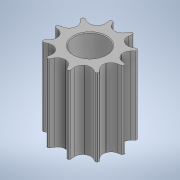
# Autodesk Inventor part: Pulley HTD 3M 10T
Saved by Autodesk Inventor 2022.2 (Build 262287030, 287C)
## iProperties
Created: 2019-06-06
Part Number: Pulley HTD 3M 10T
Material: Generic
Description: STEP AP214
Document SubType Name: Modeling
Designer: Jochen
Density: 1 g/cm^3
Appearance: Default(2)
Sending System: PARTsolutions
Title: C:/Users/StangenbergN/Desktop/Steps Zahnriemenräder/K166_HTD-Zahnwellen/17091100.stp
Revision Number: NONE
Autodesk Inventor part; units mm, degrees
ref_plane "YZ Plane" through (0, 0, 0) normal (1, 0, 0) x (0, 1, 0)
ref_plane "XZ Plane" through (0, 0, 0) normal (0, 1, 0) x (-1, 0, 0)
ref_plane "XY Plane" through (0, 0, 0) normal (0, 0, 1) x (1, 0, 0)
sketch "Sketch3" plane through (0, 0, 0) normal (0, 1, 0) x (-1, 0, 0)
  line L0 (0.8939, 3.7122) -> (1.1141, 4.1058)
  arc A0 (1.3267, 4.19) -> (1.1141, 4.1058) centre (1.272, 4.0174) ccw
  arc A1 (1.3895, 4.1696) -> (1.3267, 4.19) centre (0, 0) ccw
  arc A2 (1.512, 3.9765) -> (1.3895, 4.1696) centre (1.3323, 3.9979) ccw
  line L1 (1.512, 3.9765) -> (1.4588, 3.5286)
  arc A3 (1.4588, 3.5286) -> (1.8604, 2.6099) centre (2.4429, 3.4117) ccw
  line L2 (1.8604, 2.6099) -> (1.9073, 2.5759)
  arc A4 (1.9073, 2.5759) -> (2.9051, 2.4778) centre (2.4898, 3.3776) ccw
  line L3 (2.9051, 2.4778) -> (3.3146, 2.6668)
  arc A5 (3.5361, 2.61) -> (3.3146, 2.6668) centre (3.3905, 2.5025) ccw
  arc A6 (3.5749, 2.5565) -> (3.5361, 2.61) centre (0, 0) ccw
  arc A7 (3.5606, 2.3283) -> (3.5749, 2.5565) centre (3.4277, 2.4512) ccw
  line L4 (3.5606, 2.3283) -> (3.2543, 1.9972)
  arc A8 (3.2543, 1.9972) -> (3.0392, 1.018) centre (3.9817, 1.3242) ccw
  line L5 (3.0392, 1.018) -> (3.0571, 0.9628)
  arc A9 (3.0571, 0.9628) -> (3.8067, 0.297) centre (3.9996, 1.2691) ccw
  line L6 (3.8067, 0.297) -> (4.2491, 0.2092)
  arc A10 (4.3949, 0.033) -> (4.2491, 0.2092) centre (4.2139, 0.0317) ccw
  arc A11 (4.3949, -0.033) -> (4.3949, 0.033) centre (0, 0) ccw
  arc A12 (4.2491, -0.2092) -> (4.3949, -0.033) centre (4.2139, -0.0317) ccw
  line L7 (4.2491, -0.2092) -> (3.8067, -0.297)
  arc A13 (3.8067, -0.297) -> (3.0571, -0.9628) centre (3.9996, -1.2691) ccw
  line L8 (3.0571, -0.9628) -> (3.0392, -1.018)
  arc A14 (3.0392, -1.018) -> (3.2543, -1.9972) centre (3.9817, -1.3242) ccw
  line L9 (3.2543, -1.9972) -> (3.5606, -2.3283)
  arc A15 (3.5749, -2.5565) -> (3.5606, -2.3283) centre (3.4277, -2.4512) ccw
  arc A16 (3.5361, -2.61) -> (3.5749, -2.5565) centre (0, 0) ccw
  arc A17 (3.3146, -2.6668) -> (3.5361, -2.61) centre (3.3905, -2.5025) ccw
  line L10 (3.3146, -2.6668) -> (2.9051, -2.4778)
  arc A18 (2.9051, -2.4778) -> (1.9073, -2.5759) centre (2.4898, -3.3776) ccw
  line L11 (1.9073, -2.5759) -> (1.8604, -2.6099)
  arc A19 (1.8604, -2.6099) -> (1.4588, -3.5286) centre (2.4429, -3.4117) ccw
  line L12 (1.4588, -3.5286) -> (1.512, -3.9765)
  arc A20 (1.3895, -4.1696) -> (1.512, -3.9765) centre (1.3323, -3.9979) ccw
  arc A21 (1.3267, -4.19) -> (1.3895, -4.1696) centre (0, 0) ccw
  arc A22 (1.1141, -4.1058) -> (1.3267, -4.19) centre (1.272, -4.0174) ccw
  line L13 (1.1141, -4.1058) -> (0.8939, -3.7122)
  arc A23 (0.8939, -3.7122) -> (0.029, -3.205) centre (0.029, -4.196) ccw
  line L14 (0.029, -3.205) -> (-0.029, -3.205)
  arc A24 (-0.029, -3.205) -> (-0.8939, -3.7122) centre (-0.029, -4.196) ccw
  line L15 (-0.8939, -3.7122) -> (-1.1141, -4.1058)
  arc A25 (-1.3267, -4.19) -> (-1.1141, -4.1058) centre (-1.272, -4.0174) ccw
  arc A26 (-1.3895, -4.1696) -> (-1.3267, -4.19) centre (0, 0) ccw
  arc A27 (-1.512, -3.9765) -> (-1.3895, -4.1696) centre (-1.3323, -3.9979) ccw
  line L16 (-1.512, -3.9765) -> (-1.4588, -3.5286)
  arc A28 (-1.4588, -3.5286) -> (-1.8604, -2.6099) centre (-2.4429, -3.4117) ccw
  line L17 (-1.8604, -2.6099) -> (-1.9073, -2.5759)
  arc A29 (-1.9073, -2.5759) -> (-2.9051, -2.4778) centre (-2.4898, -3.3776) ccw
  line L18 (-2.9051, -2.4778) -> (-3.3146, -2.6668)
  arc A30 (-3.5361, -2.61) -> (-3.3146, -2.6668) centre (-3.3905, -2.5025) ccw
  arc A31 (-3.5749, -2.5565) -> (-3.5361, -2.61) centre (0, 0) ccw
  arc A32 (-3.5606, -2.3283) -> (-3.5749, -2.5565) centre (-3.4277, -2.4512) ccw
  line L19 (-3.5606, -2.3283) -> (-3.2543, -1.9972)
  arc A33 (-3.2543, -1.9972) -> (-3.0392, -1.018) centre (-3.9817, -1.3242) ccw
  line L20 (-3.0392, -1.018) -> (-3.0571, -0.9628)
  arc A34 (-3.0571, -0.9628) -> (-3.8067, -0.297) centre (-3.9996, -1.2691) ccw
  line L21 (-3.8067, -0.297) -> (-4.2491, -0.2092)
  arc A35 (-4.3949, -0.033) -> (-4.2491, -0.2092) centre (-4.2139, -0.0317) ccw
  arc A36 (-4.3949, 0.033) -> (-4.3949, -0.033) centre (0, 0) ccw
  arc A37 (-4.2491, 0.2092) -> (-4.3949, 0.033) centre (-4.2139, 0.0317) ccw
  line L22 (-4.2491, 0.2092) -> (-3.8067, 0.297)
  arc A38 (-3.8067, 0.297) -> (-3.0571, 0.9628) centre (-3.9996, 1.2691) ccw
  line L23 (-3.0571, 0.9628) -> (-3.0392, 1.018)
  arc A39 (-3.0392, 1.018) -> (-3.2543, 1.9972) centre (-3.9817, 1.3242) ccw
  line L24 (-3.2543, 1.9972) -> (-3.5606, 2.3283)
  arc A40 (-3.5749, 2.5565) -> (-3.5606, 2.3283) centre (-3.4277, 2.4512) ccw
  arc A41 (-3.5361, 2.61) -> (-3.5749, 2.5565) centre (0, 0) ccw
  arc A42 (-3.3146, 2.6668) -> (-3.5361, 2.61) centre (-3.3905, 2.5025) ccw
  line L25 (-3.3146, 2.6668) -> (-2.9051, 2.4778)
  arc A43 (-2.9051, 2.4778) -> (-1.9073, 2.5759) centre (-2.4898, 3.3776) ccw
  line L26 (-1.9073, 2.5759) -> (-1.8604, 2.6099)
  arc A44 (-1.8604, 2.6099) -> (-1.4588, 3.5286) centre (-2.4429, 3.4117) ccw
  line L27 (-1.4588, 3.5286) -> (-1.512, 3.9765)
  arc A45 (-1.3895, 4.1696) -> (-1.512, 3.9765) centre (-1.3323, 3.9979) ccw
  arc A46 (-1.3267, 4.19) -> (-1.3895, 4.1696) centre (0, 0) ccw
  arc A47 (-1.1141, 4.1058) -> (-1.3267, 4.19) centre (-1.272, 4.0174) ccw
  line L28 (-1.1141, 4.1058) -> (-0.8939, 3.7122)
  arc A48 (-0.8939, 3.7122) -> (-0.029, 3.205) centre (-0.029, 4.196) ccw
  line L29 (-0.029, 3.205) -> (0.029, 3.205)
  arc A49 (0.029, 3.205) -> (0.8939, 3.7122) centre (0.029, 4.196) ccw
  arc A50 (-0.029, -3.405) -> (-0.7193, -3.8098) centre (-0.029, -4.196) ccw
  line L30 (-0.029, -3.405) -> (0.029, -3.405)
  arc A51 (0.7193, -3.8098) -> (0.029, -3.405) centre (0.029, -4.196) ccw
  line L31 (0.7193, -3.8098) -> (0.9395, -4.2034)
  arc A52 (0.9395, -4.2034) -> (1.387, -4.3807) centre (1.272, -4.0174) ccw
  arc A53 (1.387, -4.3807) -> (1.4527, -4.3593) centre (0, 0) ccw
  arc A54 (1.4527, -4.3593) -> (1.7106, -3.9529) centre (1.3323, -3.9979) ccw
  line L32 (1.7106, -3.9529) -> (1.6574, -3.505)
  arc A55 (1.9779, -2.7717) -> (1.6574, -3.505) centre (2.4429, -3.4117) ccw
  line L33 (1.9779, -2.7717) -> (2.0249, -2.7377)
  arc A56 (2.8213, -2.6594) -> (2.0249, -2.7377) centre (2.4898, -3.3776) ccw
  line L34 (2.8213, -2.6594) -> (3.2308, -2.8484)
  arc A57 (3.2308, -2.8484) -> (3.697, -2.7287) centre (3.3905, -2.5025) ccw
  arc A58 (3.697, -2.7287) -> (3.7376, -2.6729) centre (0, 0) ccw
  arc A59 (3.7376, -2.6729) -> (3.7074, -2.1925) centre (3.4277, -2.4512) ccw
  line L35 (3.7074, -2.1925) -> (3.4011, -1.8614)
  arc A60 (3.2294, -1.0798) -> (3.4011, -1.8614) centre (3.9817, -1.3242) ccw
  line L36 (3.2294, -1.0798) -> (3.2473, -1.0246)
  arc A61 (3.8456, -0.4932) -> (3.2473, -1.0246) centre (3.9996, -1.2691) ccw
  line L37 (3.8456, -0.4932) -> (4.288, -0.4054)
  arc A62 (4.288, -0.4054) -> (4.5949, -0.0345) centre (4.2139, -0.0317) ccw
  arc A63 (4.5949, -0.0345) -> (4.5949, 0.0345) centre (0, 0) ccw
  arc A64 (4.5949, 0.0345) -> (4.288, 0.4054) centre (4.2139, 0.0317) ccw
  line L38 (4.288, 0.4054) -> (3.8456, 0.4932)
  arc A65 (3.2473, 1.0246) -> (3.8456, 0.4932) centre (3.9996, 1.2691) ccw
  line L39 (3.2473, 1.0246) -> (3.2294, 1.0798)
  arc A66 (3.4011, 1.8614) -> (3.2294, 1.0798) centre (3.9817, 1.3242) ccw
  line L40 (3.4011, 1.8614) -> (3.7074, 2.1925)
  arc A67 (3.7074, 2.1925) -> (3.7376, 2.6729) centre (3.4277, 2.4512) ccw
  arc A68 (3.7376, 2.6729) -> (3.697, 2.7287) centre (0, 0) ccw
  arc A69 (3.697, 2.7287) -> (3.2308, 2.8484) centre (3.3905, 2.5025) ccw
  line L41 (3.2308, 2.8484) -> (2.8213, 2.6594)
  arc A70 (2.0249, 2.7377) -> (2.8213, 2.6594) centre (2.4898, 3.3776) ccw
  line L42 (2.0249, 2.7377) -> (1.9779, 2.7717)
  arc A71 (1.6574, 3.505) -> (1.9779, 2.7717) centre (2.4429, 3.4117) ccw
  line L43 (1.6574, 3.505) -> (1.7106, 3.9529)
  arc A72 (1.7106, 3.9529) -> (1.4527, 4.3593) centre (1.3323, 3.9979) ccw
  arc A73 (1.4527, 4.3593) -> (1.387, 4.3807) centre (0, 0) ccw
  arc A74 (1.387, 4.3807) -> (0.9395, 4.2034) centre (1.272, 4.0174) ccw
  line L44 (0.9395, 4.2034) -> (0.7193, 3.8098)
  arc A75 (0.029, 3.405) -> (0.7193, 3.8098) centre (0.029, 4.196) ccw
  line L45 (0.029, 3.405) -> (-0.029, 3.405)
  arc A76 (-0.7193, 3.8098) -> (-0.029, 3.405) centre (-0.029, 4.196) ccw
  line L46 (-0.7193, 3.8098) -> (-0.9395, 4.2034)
  arc A77 (-0.9395, 4.2034) -> (-1.387, 4.3807) centre (-1.272, 4.0174) ccw
  arc A78 (-1.387, 4.3807) -> (-1.4527, 4.3593) centre (0, 0) ccw
  arc A79 (-1.4527, 4.3593) -> (-1.7106, 3.9529) centre (-1.3323, 3.9979) ccw
  line L47 (-1.7106, 3.9529) -> (-1.6574, 3.505)
  arc A80 (-1.9779, 2.7717) -> (-1.6574, 3.505) centre (-2.4429, 3.4117) ccw
  line L48 (-1.9779, 2.7717) -> (-2.0249, 2.7377)
  arc A81 (-2.8213, 2.6594) -> (-2.0249, 2.7377) centre (-2.4898, 3.3776) ccw
  line L49 (-2.8213, 2.6594) -> (-3.2308, 2.8484)
  arc A82 (-3.2308, 2.8484) -> (-3.697, 2.7287) centre (-3.3905, 2.5025) ccw
  arc A83 (-3.697, 2.7287) -> (-3.7376, 2.6729) centre (0, 0) ccw
  arc A84 (-3.7376, 2.6729) -> (-3.7074, 2.1925) centre (-3.4277, 2.4512) ccw
  line L50 (-3.7074, 2.1925) -> (-3.4011, 1.8614)
  arc A85 (-3.2294, 1.0798) -> (-3.4011, 1.8614) centre (-3.9817, 1.3242) ccw
  line L51 (-3.2294, 1.0798) -> (-3.2473, 1.0246)
  arc A86 (-3.8456, 0.4932) -> (-3.2473, 1.0246) centre (-3.9996, 1.2691) ccw
  line L52 (-3.8456, 0.4932) -> (-4.288, 0.4054)
  arc A87 (-4.288, 0.4054) -> (-4.5949, 0.0345) centre (-4.2139, 0.0317) ccw
  arc A88 (-4.5949, 0.0345) -> (-4.5949, -0.0345) centre (0, 0) ccw
  arc A89 (-4.5949, -0.0345) -> (-4.288, -0.4054) centre (-4.2139, -0.0317) ccw
  line L53 (-4.288, -0.4054) -> (-3.8456, -0.4932)
  arc A90 (-3.2473, -1.0246) -> (-3.8456, -0.4932) centre (-3.9996, -1.2691) ccw
  line L54 (-3.2473, -1.0246) -> (-3.2294, -1.0798)
  arc A91 (-3.4011, -1.8614) -> (-3.2294, -1.0798) centre (-3.9817, -1.3242) ccw
  line L55 (-3.4011, -1.8614) -> (-3.7074, -2.1925)
  arc A92 (-2.0249, -2.7377) -> (-2.8213, -2.6594) centre (-2.4898, -3.3776) ccw
  line L56 (-2.0249, -2.7377) -> (-1.9779, -2.7717)
  arc A93 (-1.6574, -3.505) -> (-1.9779, -2.7717) centre (-2.4429, -3.4117) ccw
  line L57 (-1.6574, -3.505) -> (-1.7106, -3.9529)
  arc A94 (-1.7106, -3.9529) -> (-1.4527, -4.3593) centre (-1.3323, -3.9979) ccw
  arc A95 (-1.4527, -4.3593) -> (-1.387, -4.3807) centre (0, 0) ccw
  arc A96 (-1.387, -4.3807) -> (-0.9395, -4.2034) centre (-1.272, -4.0174) ccw
  line L58 (-0.9395, -4.2034) -> (-0.7193, -3.8098)
  circle A97 centre (0, 0) radius 2.075
  arc A98 (-0.029, -3.455) -> (-0.6757, -3.8342) centre (-0.029, -4.196) ccw
  line L59 (-0.029, -3.455) -> (0.029, -3.455)
  arc A99 (0.6757, -3.8342) -> (0.029, -3.455) centre (0.029, -4.196) ccw
  line L60 (0.6757, -3.8342) -> (0.8959, -4.2279)
  arc A100 (0.8959, -4.2279) -> (1.4021, -4.4283) centre (1.272, -4.0174) ccw
  arc A101 (1.4021, -4.4283) -> (1.4685, -4.4067) centre (0, 0) ccw
  arc A102 (1.4685, -4.4067) -> (1.7603, -3.947) centre (1.3323, -3.9979) ccw
  line L61 (1.7603, -3.947) -> (1.7071, -3.4991)
  arc A103 (2.0073, -2.8122) -> (1.7071, -3.4991) centre (2.4429, -3.4117) ccw
  line L62 (2.0073, -2.8122) -> (2.0543, -2.7781)
  arc A104 (2.8003, -2.7048) -> (2.0543, -2.7781) centre (2.4898, -3.3776) ccw
  line L63 (2.8003, -2.7048) -> (3.2099, -2.8938)
  arc A105 (3.2099, -2.8938) -> (3.7373, -2.7584) centre (3.3905, -2.5025) ccw
  arc A106 (3.7373, -2.7584) -> (3.7783, -2.7019) centre (0, 0) ccw
  arc A107 (3.7783, -2.7019) -> (3.7441, -2.1585) centre (3.4277, -2.4512) ccw
  line L64 (3.7441, -2.1585) -> (3.4378, -1.8274)
  arc A108 (3.2769, -1.0952) -> (3.4378, -1.8274) centre (3.9817, -1.3242) ccw
  line L65 (3.2769, -1.0952) -> (3.2949, -1.0401)
  arc A109 (3.8554, -0.5422) -> (3.2949, -1.0401) centre (3.9996, -1.2691) ccw
  line L66 (3.8554, -0.5422) -> (4.2978, -0.4544)
  arc A110 (4.2978, -0.4544) -> (4.6449, -0.0349) centre (4.2139, -0.0317) ccw
  arc A111 (4.6449, -0.0349) -> (4.6449, 0.0349) centre (0, 0) ccw
  arc A112 (4.6449, 0.0349) -> (4.2978, 0.4544) centre (4.2139, 0.0317) ccw
  line L67 (4.2978, 0.4544) -> (3.8554, 0.5422)
  arc A113 (3.2949, 1.0401) -> (3.8554, 0.5422) centre (3.9996, 1.2691) ccw
  line L68 (3.2949, 1.0401) -> (3.2769, 1.0952)
  arc A114 (3.4378, 1.8274) -> (3.2769, 1.0952) centre (3.9817, 1.3242) ccw
  line L69 (3.4378, 1.8274) -> (3.7441, 2.1585)
  arc A115 (3.7441, 2.1585) -> (3.7783, 2.7019) centre (3.4277, 2.4512) ccw
  arc A116 (3.7783, 2.7019) -> (3.7373, 2.7584) centre (0, 0) ccw
  arc A117 (3.7373, 2.7584) -> (3.2099, 2.8938) centre (3.3905, 2.5025) ccw
  line L70 (3.2099, 2.8938) -> (2.8003, 2.7048)
  arc A118 (2.0543, 2.7781) -> (2.8003, 2.7048) centre (2.4898, 3.3776) ccw
  line L71 (2.0543, 2.7781) -> (2.0073, 2.8122)
  arc A119 (1.7071, 3.4991) -> (2.0073, 2.8122) centre (2.4429, 3.4117) ccw
  line L72 (1.7071, 3.4991) -> (1.7603, 3.947)
  arc A120 (1.7603, 3.947) -> (1.4685, 4.4067) centre (1.3323, 3.9979) ccw
  arc A121 (1.4685, 4.4067) -> (1.4021, 4.4283) centre (0, 0) ccw
  arc A122 (1.4021, 4.4283) -> (0.8959, 4.2279) centre (1.272, 4.0174) ccw
  line L73 (0.8959, 4.2279) -> (0.6757, 3.8342)
  arc A123 (0.029, 3.455) -> (0.6757, 3.8342) centre (0.029, 4.196) ccw
  line L74 (0.029, 3.455) -> (-0.029, 3.455)
  arc A124 (-0.6757, 3.8342) -> (-0.029, 3.455) centre (-0.029, 4.196) ccw
  line L75 (-0.6757, 3.8342) -> (-0.8959, 4.2279)
  arc A125 (-0.8959, 4.2279) -> (-1.4021, 4.4283) centre (-1.272, 4.0174) ccw
  arc A126 (-1.4021, 4.4283) -> (-1.4685, 4.4067) centre (0, 0) ccw
  arc A127 (-1.4685, 4.4067) -> (-1.7603, 3.947) centre (-1.3323, 3.9979) ccw
  line L76 (-1.7603, 3.947) -> (-1.7071, 3.4991)
  arc A128 (-2.0073, 2.8122) -> (-1.7071, 3.4991) centre (-2.4429, 3.4117) ccw
  line L77 (-2.0073, 2.8122) -> (-2.0543, 2.7781)
  arc A129 (-2.8003, 2.7048) -> (-2.0543, 2.7781) centre (-2.4898, 3.3776) ccw
  line L78 (-2.8003, 2.7048) -> (-3.2099, 2.8938)
  arc A130 (-3.2099, 2.8938) -> (-3.7373, 2.7584) centre (-3.3905, 2.5025) ccw
  arc A131 (-3.7373, 2.7584) -> (-3.7783, 2.7019) centre (0, 0) ccw
  arc A132 (-3.7783, 2.7019) -> (-3.7441, 2.1585) centre (-3.4277, 2.4512) ccw
  line L79 (-3.7441, 2.1585) -> (-3.4378, 1.8274)
  arc A133 (-3.2769, 1.0952) -> (-3.4378, 1.8274) centre (-3.9817, 1.3242) ccw
  line L80 (-3.2769, 1.0952) -> (-3.2949, 1.0401)
  arc A134 (-3.8554, 0.5422) -> (-3.2949, 1.0401) centre (-3.9996, 1.2691) ccw
  line L81 (-3.8554, 0.5422) -> (-4.2978, 0.4544)
  arc A135 (-4.2978, 0.4544) -> (-4.6449, 0.0349) centre (-4.2139, 0.0317) ccw
  arc A136 (-4.6449, 0.0349) -> (-4.6449, -0.0349) centre (0, 0) ccw
  arc A137 (-4.6449, -0.0349) -> (-4.2978, -0.4544) centre (-4.2139, -0.0317) ccw
  line L82 (-4.2978, -0.4544) -> (-3.8554, -0.5422)
  arc A138 (-3.2949, -1.0401) -> (-3.8554, -0.5422) centre (-3.9996, -1.2691) ccw
  line L83 (-3.2949, -1.0401) -> (-3.2769, -1.0952)
  arc A139 (-3.4378, -1.8274) -> (-3.2769, -1.0952) centre (-3.9817, -1.3242) ccw
  line L84 (-3.4378, -1.8274) -> (-3.7441, -2.1585)
  arc A140 (-2.0543, -2.7781) -> (-2.8003, -2.7048) centre (-2.4898, -3.3776) ccw
  line L85 (-2.0543, -2.7781) -> (-2.0073, -2.8122)
  arc A141 (-1.7071, -3.4991) -> (-2.0073, -2.8122) centre (-2.4429, -3.4117) ccw
  line L86 (-1.7071, -3.4991) -> (-1.7603, -3.947)
  arc A142 (-1.7603, -3.947) -> (-1.4685, -4.4067) centre (-1.3323, -3.9979) ccw
  arc A143 (-1.4685, -4.4067) -> (-1.4021, -4.4283) centre (0, 0) ccw
  arc A144 (-1.4021, -4.4283) -> (-0.8959, -4.2279) centre (-1.272, -4.0174) ccw
  line L87 (-0.8959, -4.2279) -> (-0.6757, -3.8342)
  point P0 (0, 0)
  dimension "d7" = 0.2
  dimension "d9" = 4.15
  dimension "d10" = 0.25
  constraints: 288 point on circle, 176 end point, 145 centre point, 148 other
  measures "d7" radial gap between concentric circles of A24 A50
  measures "d9" diameter of A97
  measures "d10" radial gap between concentric circles of A24 A98
extrude "Extrusion2" add sketch "Sketch3" along normal blind 10
chamfer "Chamfer2" distance 0.1 angle 45 2 edges at (2.075, 10, 0) (2.075, 0, 0)
body "Solid2"
body "Solid3"
